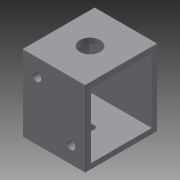
# Autodesk Inventor part: Solenoid_shell
Saved by Autodesk Inventor 2015 (Build 190159000, 159)
## iProperties
Created: 2015-11-10
Part Number: Solenoid_shell
Material: Generic
Document SubType Name: Modeling
Designer: Lauszus
Density: 1 g/cm^3
Appearance: Default
Author: Lauszus
Autodesk Inventor part; units mm, degrees
ref_plane "YZ Plane" through (0, 0, 0) normal (1, 0, 0) x (0, 1, 0)
ref_plane "XZ Plane" through (0, 0, 0) normal (0, 1, 0) x (-1, 0, 0)
ref_plane "XY Plane" through (0, 0, 0) normal (0, 0, 1) x (1, 0, 0)
sketch "Sketch1" plane through (0, 0, 0) normal (0, 1, 0) x (-1, 0, 0)
  line L0 (11.5005, 11.58) -> (-10.5995, 11.58)
  line L1 (-10.5995, 11.58) -> (-10.5995, -15.22)
  line L2 (-10.5995, -15.22) -> (11.5005, -15.22)
  line L3 (11.5005, -15.22) -> (11.5005, 11.58)
  point P0 (0, 0)
  dimension "d0" = 22.1
  dimension "d1" = 26.8
  constraints: 8 end point, 2 parallel, 1 horizontal, 1 perpendicular
  measures "d0" distance of L0.start L0.end
  measures "d1" distance of L0.end L1.end
extrude "Extrusion1" add sketch "Sketch1" along normal blind 25.4
shell "Shell1" thickness 2 removed faces 2 at (-11.5005, 8.4667, -6.2867) at (10.5995, 8.4667, 2.6466)
sketch "Sketch2" plane through (0, 0, 0) normal (0, -1, 0) x (1, 0, 0)
  line L0 (-11.5005, 11.58) -> (10.5995, 11.58) projected
  line L1 (-0.4505, 11.58) -> (-0.4505, -15.22)
  line L2 (10.5995, -15.22) -> (-11.5005, -15.22) projected
  circle A0 centre (-0.4505, -1.82) radius 9.5
  circle A1 centre (-6.4505, 5.5454) radius 1.5
  circle A2 centre (5.5495, -9.1855) radius 1.5
  point P0 (0, 0)
  dimension "d4" = 19
  dimension "d5" = 3
  dimension "d6" = 3
  dimension "d7" = 6
  dimension "d8" = 12
  constraints: 3 centre point, 3 midpoint, 2 end point, 2 point on circle
  measures "d4" diameter of A0
  measures "d5" diameter of A1
  measures "d6" diameter of A2
  measures "d7" distance from line of L1 A1.centre
  measures "d8" horizontal distance of A2.centre A1.centre
extrude "Extrusion2" cut sketch "Sketch2" against normal up to next contours A1 A0 | A0 A1 | A2 A0 | A0 A2
sketch "Sketch3" plane through (-11.5005, 0, 11.58) normal (0, 0, 1) x (1, 0, 0)
  line L0 (22.1, 0) -> (0, 0) projected
  line L1 (11.05, 0) -> (11.05, 25.4)
  line L2 (0, 25.4) -> (22.1, 25.4) projected
  circle A0 centre (11.05, 12.7) radius 3.6
  point P0 (11.5005, 0)
  dimension "d12" = 7.2
  constraints: 3 midpoint, 2 end point, 1 centre point
  measures "d12" diameter of A0
extrude "Extrusion3" cut sketch "Sketch3" against normal up to next
sketch "Sketch4" plane through (10.5995, 0, -15.22) normal (0, 0, -1) x (-1, 0, 0)
  line L0 (0, 25.4) -> (22.1, 25.4) projected
  line L1 (11.05, 25.4) -> (11.05, 0)
  line L2 (22.1, 0) -> (0, 0) projected
  circle A0 centre (11.05, 12.7) radius 1.5
  point P0 (10.5995, 0)
  dimension "d15" = 3
  constraints: 3 midpoint, 2 end point, 1 centre point
  measures "d15" diameter of A0
extrude "Extrusion4" cut sketch "Sketch4" against normal up to next
fillet "Fillet1" radius 0.2 16 edges at (-11.5005, 12.7, 11.58) (-0.4505, 0, 11.58) (10.5995, 12.7, 11.58) (10.5995, 0, -1.82) (-11.5005, 0, -1.82) (-0.4505, 0, -15.22) (10.5995, 12.7, -15.22) (-11.5005, 12.7, -15.22) (-0.4505, 25.4, -15.22) (-11.5005, 25.4, -1.82) (-0.4505, 25.4, 11.58) (10.5995, 25.4, -1.82) (-11.5005, 12.7, -13.22) (-11.5005, 2, -1.82) (-11.5005, 12.7, 9.58) (-11.5005, 23.4, -1.82)
body "Solid1"
